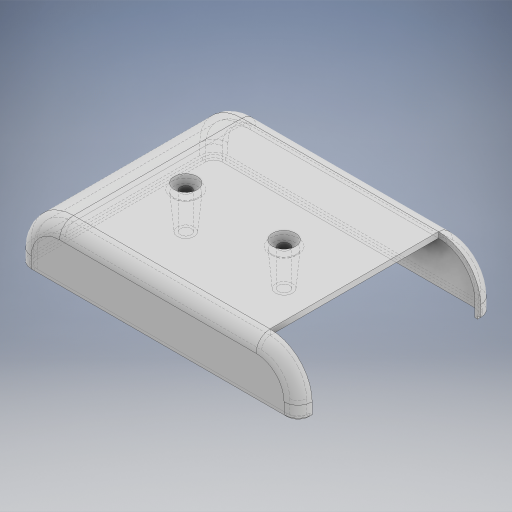
# Autodesk Inventor part: A1.1
Saved by Autodesk Inventor 2024 (Build 280153000, 153)
## iProperties
Created: 2024-01-30
Part Number: A1.1
Material: Generic
Document SubType Name: Modeling
Designer: Alex
Density: 1 g/cm^3
Appearance: Default
Author: Alex
Autodesk Inventor part; units mm, degrees
note: some values were not read from the file. Chosen so that the rebuilt part matches the saved one: direction of "Hole1"; direction of "Hole2".
ref_plane "YZ Plane" through (0, 0, 0) normal (1, 0, 0) x (0, 1, 0)
ref_plane "XZ Plane" through (0, 0, 0) normal (0, 1, 0) x (-1, 0, 0)
sketch "Sketch1" plane through (0, 0, 0) normal (0, 1, 0) x (-1, 0, 0)
  line L0 (0, 0) -> (100, 0)
  line L1 (100, 0) -> (100, -70)
  line L2 (100, -70) -> (0, -70)
  line L3 (0, -70) -> (0, 0)
  dimension "d0" = 100
  dimension "d1" = 70
  constraints: 8 end point, 2 parallel, 1 horizontal, 1 perpendicular
  measures "d0" distance of L1.end L2.end
  measures "d1" distance of L0.end L1.end
extrude "Extrusion1" add sketch "Sketch1" along normal blind 20
fillet "Fillet1" radius 15 2 edges at (-100, 20, -35) (0, 20, -35)
fillet "Fillet2" radius 5 10 edges at (-4.3934, 15.6066, 0) (0, 2.5, 0) (-95.6066, 15.6066, 0) (-100, 2.5, 0) (-50, 20, 0) (-95.6066, 15.6066, -70) (-100, 2.5, -70) (-4.3934, 15.6066, -70) (0, 2.5, -70) (-50, 20, -70)
shell "Shell1" thickness 2 removed faces 3 at (-0.0419, 6.121, -45) at (0, 1.6667, -25) at (-65, 0, -46.6667)
ref_plane "Work Plane1" through (0, 5, 0) normal (0, 1, 0) x (1, 0, 0)
sketch "Sketch2" plane through (0, 5, 0) normal (0, 1, 0) x (1, 0, 0)
  line L0 (-85, 65) -> (-15, 65) construction
  line L1 (-15, 65) -> (-15, 5) construction
  line L2 (-15, 5) -> (-85, 5) construction
  line L3 (-85, 5) -> (-85, 65) construction
  line L4 (-85, 5) -> (-85, 65) construction
  line L5 (-85, 35) -> (-15, 35) construction
  line L6 (-85, 35) -> (-75, 35) construction
  line L7 (-75, 35) -> (-75, 65) construction
  line L8 (-100, 65) -> (-100, 5) construction
  line L9 (-98, 65) -> (-98, 5) construction
  line L10 (-5, 70) -> (-95, 70) construction
  line L11 (-5, 68) -> (-95, 68) construction
  line L12 (-95, 2) -> (-5, 2) construction
  line L13 (-95, 0) -> (-5, 0) construction
  line L14 (-40, 35) -> (-40, 65) construction
  circle A0 centre (-75, 35) radius 3
  circle A1 centre (-40, 35) radius 3
  point P0 (0, 0)
  dimension "d9" = 25
  dimension "d10" = 35
  dimension "d11" = 6
  dimension "d12" = 6
  constraints: 8 end point, 4 point on line, 3 perpendicular, 2 centre point, 2 coincident, 2 midpoint
  measures "d9" distance between parallel lines of L7 L8
  measures "d10" distance between parallel lines of L7 L14
  measures "d11" diameter of A0
  measures "d12" diameter of A1
extrude "Extrusion2" add sketch "Sketch2" along normal up to surface (13 mm away) draft 5
sketch "Sketch3" plane through (0, 20, 0) normal (0, 1, 0) x (1, 0, 0)
  circle A0 centre (-75, 35) radius 3 construction
  circle A1 centre (-75, 35) radius 4.1374 construction
  circle A2 centre (-40, 35) radius 3 construction
  circle A3 centre (-40, 35) radius 4.1374 construction
  line L0 (-85, 65) -> (-15, 65) construction
  line L1 (-85, 5) -> (-85, 65) construction
  line L2 (-15, 5) -> (-85, 5) construction
  line L3 (-15, 65) -> (-15, 5) construction
  point P0 (0, 0)
hole "Hole1" at (-75, 20, -35) direction (0, -1, 0) diameter 3.9 depth 15 countersink diameter 8.2 countersink angle 90
hole "Hole2" at (-40, 20, -35) direction (0, -1, 0) diameter 3.9 depth 15 countersink diameter 8.2 countersink angle 90
fillet "Fillet3" radius 1 2 edges at (-44.1374, 18, -35) (-79.1374, 18, -35)
sketch "Sketch4" plane through (0, 0, 0) normal (0, -1, 0) x (1, 0, 0)
  arc A0 (0, -5) -> (-5, 0) centre (-5, -5) ccw projected
  line L0 (-95, 0) -> (-5, 0) projected
  arc A1 (-95, 0) -> (-100, -5) centre (-95, -5) ccw projected
  line L1 (-100, -65) -> (-100, -5) projected
  arc A2 (-100, -65) -> (-95, -70) centre (-95, -65) ccw projected
  line L2 (-5, -70) -> (-95, -70) projected
  arc A3 (-5, -70) -> (0, -65) centre (-5, -65) ccw projected
  arc A4 (-1, -5) -> (-5, -1) centre (-5, -5) ccw
  line L3 (-5, -1) -> (-95, -1)
  arc A5 (-95, -1) -> (-99, -5) centre (-95, -5) ccw
  line L4 (-99, -5) -> (-99, -65)
  arc A6 (-99, -65) -> (-95, -69) centre (-95, -65) ccw
  line L5 (-95, -69) -> (-5, -69)
  arc A7 (-5, -69) -> (-1, -65) centre (-5, -65) ccw
  line L6 (-2, -5) -> (0, -5) projected
  line L7 (-1, -5) -> (0, -5)
  line L8 (0, -65) -> (-2, -65) projected
  line L9 (-1, -65) -> (0, -65)
  point P0 (0, 0)
  dimension "d30" = 1
  constraints: 10 end point, 8 point on circle, 4 centre point, 2 collinear, 6 other
  measures "d30" radial gap between concentric circles of A0 A4
extrude "Extrusion3" cut sketch "Sketch4" against normal blind 1
body "Solid1"
